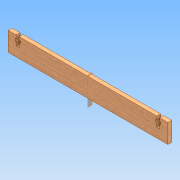
# Autodesk Inventor part: Selection_Ramp 1_Mid piece
Saved by Autodesk Inventor 2018.1 (Build 221171000, 171)
## iProperties
Created: 2019-02-07
Part Number: Selection_Ramp 1_Mid piece
Material: Wood (Cherry)
Document SubType Name: Modeling
Designer: James
Density: 0.63 g/cm^3
Appearance: Cherry - Natural Low Gloss
Author: James
Autodesk Inventor part; units mm, degrees
ref_plane "YZ Plane" through (0, 0, 0) normal (1, 0, 0) x (0, 1, 0)
ref_plane "XZ Plane" through (0, 0, 0) normal (0, 1, 0) x (-1, 0, 0)
ref_plane "XY Plane" through (0, 0, 0) normal (0, 0, 1) x (1, 0, 0)
sketch "Sketch3" plane through (0, 0, 0) normal (0, 1, 0) x (-1, 0, 0)
  line L0 (0, 0) -> (250, 0)
  line L1 (250, 0) -> (250, -30)
  line L2 (250, -30) -> (0, -30)
  line L3 (0, -30) -> (0, 0)
  dimension "d24" = 250
  dimension "d25" = 30
  constraints: 8 end point, 2 parallel, 1 horizontal, 1 perpendicular
  measures "d24" distance of L1.end L2.end
  measures "d25" distance of L0.end L1.end
extrude "Extrusion2" add sketch "Sketch3" along normal blind 6
sketch "Sketch4" plane through (0, 6, 0) normal (0, 1, 0) x (1, 0, 0)
  line L0 (-250, 0) -> (0, 0) projected
  line L1 (-17.25, 0) -> (-12.75, 0)
  line L2 (-12.75, 0) -> (-12.75, 15)
  line L3 (-12.75, 15) -> (-17.25, 15)
  line L4 (-17.25, 15) -> (-17.25, 0)
  line L5 (-19, 5) -> (-11, 5)
  line L6 (-11, 5) -> (-11, 9)
  line L7 (-11, 9) -> (-19, 9)
  line L8 (-19, 9) -> (-19, 5)
  line L9 (0, 0) -> (0, 30) projected
  point P0 (-15, 9)
  point P1 (-15, 15)
  dimension "d28" = 4.5
  dimension "d29" = 15
  dimension "d30" = 8
  dimension "d31" = 5
  dimension "d32" = 4
  dimension "d33" = 12.75
  constraints: 16 end point, 4 parallel, 2 horizontal, 2 midpoint, 2 perpendicular, 1 horizontal alignment, 1 point on line, 1 vertical alignment
  measures "d28" distance between parallel lines of L4 L2
  measures "d29" distance of L1.end L2.end
  measures "d30" distance of L5.start L5.end
  measures "d31" distance between parallel lines of L0 L5
  measures "d32" distance of L7.end L5.start
  measures "d33" distance between parallel lines of L2 L9
extrude "Extrusion3" cut sketch "Sketch4" against normal through all
ref_plane "Work Plane13" through (-125, 0, 0) normal (1, 0, 0) x (0, 0, -1)
mirror "Mirror1" about plane through (-125, 0, 0) normal (1, 0, 0) of "Extrusion3"
body "Solid2"
